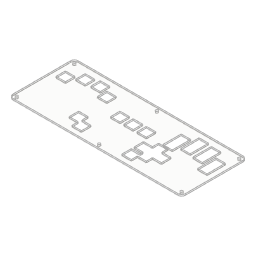
HTangl V2 Top Panel (Autodesk Fusion 360 design; units mm, degrees)
Autodesk Fusion 360 part; units mm, degrees
sketch "Refrence" plane through (0, 0, 0) normal (0, 0, 1) x (1, 0, 0)
  line L0 (183.2, 69.2) -> (-183.2, 69.2)
  line L1 (-183.2, 69.2) -> (-183.2, -69.2)
  line L2 (-183.2, -69.2) -> (183.2, -69.2)
  line L3 (183.2, -69.2) -> (183.2, 69.2)
  dimension "d1" = 366.4
  dimension "d2" = 138.4
  constraint horizontal L0
  constraint perpendicular L0 L1
  constraint parallel L0 L2
  constraint parallel L1 L3
  measures "d1" distance of L1.end L2.end
  measures "d2" distance of L0.end L1.end
sketch "Top Panel" plane through (0, 0, 0) normal (0, 0, 1) x (1, 0, 0)
  line L0 (150, 37) -> (170, 37)
  line L1 (170, -2) -> (150, -2)
  line L2 (124, 14) -> (144, 14)
  line L3 (144, 53) -> (124, 53)
  line L4 (115, 56) -> (95, 56)
  line L5 (95, 17) -> (115, 17)
  line L6 (69, 44) -> (89, 44)
  line L7 (89, 5) -> (69, 5)
  line L8 (62, 3) -> (82, 3)
  line L9 (82, 3) -> (82, -10)
  line L10 (62, -10) -> (62, 3)
  line L11 (43, -10) -> (62, -10)
  line L12 (62, -30) -> (43, -30)
  line L13 (43, -30) -> (43, -10)
  line L14 (82, -30) -> (82, -43)
  line L15 (82, -43) -> (63, -43)
  line L16 (62, -36) -> (62, -30)
  line L17 (82, -10) -> (101, -10)
  line L18 (101, -10) -> (101, -30)
  line L19 (101, -30) -> (82, -30)
  line L20 (43, -36) -> (62, -36)
  line L21 (63, -43) -> (63, -56)
  line L22 (63, -56) -> (43, -56)
  line L23 (43, -56) -> (43, -36)
  line L24 (18, 21) -> (38, 21)
  line L25 (38, 21) -> (38, 1)
  line L26 (38, 1) -> (18, 1)
  line L27 (18, 1) -> (18, 21)
  line L28 (-10, 21) -> (10, 21)
  line L29 (10, 21) -> (10, 1)
  line L30 (10, 1) -> (-10, 1)
  line L31 (-10, 1) -> (-10, 21)
  line L32 (-38, 21) -> (-18, 21)
  line L33 (-18, 21) -> (-18, 1)
  line L34 (-18, 1) -> (-38, 1)
  line L35 (-38, 1) -> (-38, 21)
  line L36 (-62, -36) -> (-43, -36)
  line L37 (-43, -36) -> (-43, -56)
  line L38 (-43, -56) -> (-63, -56)
  line L39 (-63, -56) -> (-63, -43)
  line L40 (-82, -23) -> (-62, -23)
  line L41 (-62, -23) -> (-62, -36)
  line L42 (-63, -43) -> (-82, -43)
  line L43 (-82, -43) -> (-82, -23)
  line L44 (-89, 44) -> (-69, 44)
  line L45 (-69, 44) -> (-69, 24)
  line L46 (-69, 24) -> (-89, 24)
  line L47 (-89, 24) -> (-89, 44)
  line L48 (-115, 56) -> (-95, 56)
  line L49 (-95, 56) -> (-95, 36)
  line L50 (-95, 36) -> (-115, 36)
  line L51 (-115, 36) -> (-115, 56)
  line L52 (-144, 53) -> (-124, 53)
  line L53 (-124, 53) -> (-124, 33)
  line L54 (-124, 33) -> (-144, 33)
  line L55 (-144, 33) -> (-144, 53)
  line L56 (-170, 37) -> (-150, 37)
  line L57 (-150, 37) -> (-150, 17)
  line L58 (-150, 17) -> (-170, 17)
  line L59 (-170, 17) -> (-170, 37)
  line L60 (69, 44) -> (69, 5)
  line L61 (89, 5) -> (89, 44)
  line L62 (95, 56) -> (95, 17)
  line L63 (115, 56) -> (115, 17)
  line L64 (124, 53) -> (124, 14)
  line L65 (144, 53) -> (144, 14)
  line L66 (150, 37) -> (150, -2)
  line L67 (170, 37) -> (170, -2)
  line L68 (175.2, 69.2) -> (-175.2, 69.2)
  line L69 (-183.2, 61.2) -> (-183.2, -61.2)
  line L70 (-175.2, -69.2) -> (175.2, -69.2)
  line L71 (183.2, -61.2) -> (183.2, 61.2)
  arc A0 (-175.2, 69.2) -> (-183.2, 61.2) centre (-175.2, 61.2) ccw
  arc A1 (183.2, 61.2) -> (175.2, 69.2) centre (175.2, 61.2) ccw
  arc A2 (175.2, -69.2) -> (183.2, -61.2) centre (175.2, -61.2) ccw
  arc A3 (-183.2, -61.2) -> (-175.2, -69.2) centre (-175.2, -61.2) ccw
  circle A4 centre (0, 61.2) radius 2.6
  circle A5 centre (-175.2, 61.2) radius 2.6
  circle A6 centre (-175.2, -61.2) radius 2.6
  circle A7 centre (0, -61.2) radius 2.6
  circle A8 centre (175.2, -61.2) radius 2.6
  circle A9 centre (175.2, 61.2) radius 2.6
  point P0 (160, 27)
  point P1 (160, 8)
  point P2 (134, 24)
  point P3 (134, 43)
  point P4 (105, 46)
  point P5 (105, 27)
  point P6 (79, 34)
  point P7 (79, 15)
  point P8 (72, -7)
  point P9 (53, -20)
  point P10 (72, -33)
  point P11 (91, -20)
  point P12 (53, -46)
  point P13 (28, 11)
  point P14 (0, 11)
  point P15 (-28, 11)
  point P16 (-53, -46)
  point P17 (-72, -33)
  point P18 (-79, 34)
  point P19 (-105, 46)
  point P20 (-134, 43)
  point P21 (-160, 27)
  dimension "d3" = 8
  dimension "d6" = 5.2
  dimension "d7" = 5.2
  dimension "d8" = 5.2
  dimension "d9" = 5.2
  dimension "d10" = 5.2
  dimension "d11" = 5.2
  constraint horizontal L0
  constraint horizontal L2
  constraint horizontal L6
  constraint horizontal L8
  constraint perpendicular L8 L9
  constraint parallel L9 L10
  constraint horizontal L11
  constraint parallel L11 L12
  constraint parallel L14 L16
  constraint horizontal L17
  constraint perpendicular L17 L18
  constraint parallel L17 L19
  constraint horizontal L20
  constraint perpendicular L20 L21
  constraint parallel L20 L22
  constraint parallel L21 L23
  constraint horizontal L24
  constraint perpendicular L24 L25
  constraint parallel L24 L26
  constraint parallel L25 L27
  constraint horizontal L28
  constraint perpendicular L28 L29
  constraint parallel L28 L30
  constraint parallel L29 L31
  constraint horizontal L32
  constraint perpendicular L32 L33
  constraint parallel L32 L34
  constraint parallel L33 L35
  constraint horizontal L36
  constraint perpendicular L36 L37
  constraint parallel L36 L38
  constraint parallel L37 L39
  constraint horizontal L40
  constraint perpendicular L40 L41
  constraint parallel L40 L42
  constraint parallel L41 L43
  constraint horizontal L44
  constraint perpendicular L44 L45
  constraint parallel L44 L46
  constraint parallel L45 L47
  constraint horizontal L48
  constraint perpendicular L48 L49
  constraint parallel L48 L50
  constraint parallel L49 L51
  constraint horizontal L52
  constraint perpendicular L52 L53
  constraint parallel L52 L54
  constraint parallel L53 L55
  constraint horizontal L56
  constraint perpendicular L56 L57
  constraint parallel L56 L58
  constraint parallel L57 L59
  constraint perpendicular L7 L60
  constraint perpendicular L6 L61
  constraint perpendicular L5 L62
  constraint perpendicular L5 L63
  constraint perpendicular L3 L64
  constraint perpendicular L2 L65
  constraint perpendicular L1 L66
  constraint perpendicular L1 L67
  constraint horizontal L68
  constraint perpendicular L68 L69
  constraint parallel L68 L70
  constraint parallel L69 L71
  constraint tangent L68 A0
  constraint tangent L69 A0
  constraint tangent L68 A1
  constraint tangent L71 A1
  constraint equal A0 A1
  constraint tangent L70 A2
  constraint tangent L71 A2
  constraint equal A0 A2
  constraint tangent L69 A3
  constraint tangent L70 A3
  constraint equal A0 A3
  constraint concentric A0 A5
  constraint concentric A3 A6
  constraint concentric A2 A8
  constraint concentric A1 A9
  measures "d3" radius of A0
  measures "d6" diameter of A4
  measures "d7" diameter of A5
  measures "d8" diameter of A6
  measures "d9" diameter of A7
  measures "d10" diameter of A8
  measures "d11" diameter of A9
extrude "Extrude1" add sketch "Top Panel" along normal blind 3
